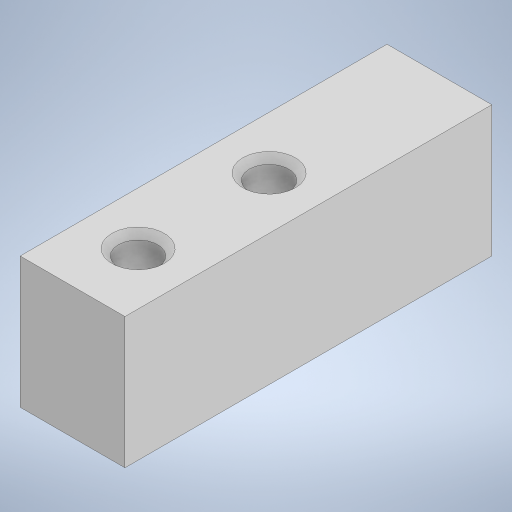
# Autodesk Inventor part: Ограничитель
Saved by Autodesk Inventor 2023 (Build 270158000, 158)
## iProperties
Created: 2022-05-17
Part Number: Ограничитель
Material: Типовые
Document SubType Name: Modeling
Designer: avkap
Density: 1 g/cm^3
Appearance: По умолчанию
Author: avkap
Autodesk Inventor part; units mm, degrees
ref_plane "YZ Plane" through (0, 0, 0) normal (1, 0, 0) x (0, 1, 0)
ref_plane "XZ Plane" through (0, 0, 0) normal (0, 1, 0) x (-1, 0, 0)
ref_plane "XY Plane" through (0, 0, 0) normal (0, 0, 1) x (1, 0, 0)
sketch "Эскиз1" plane through (0, 0, 0) normal (0, 1, 0) x (-1, 0, 0)
  line L0 (0, 0) -> (-8, 0)
  line L1 (-8, 0) -> (-8, -28)
  line L2 (-8, -28) -> (0, -28)
  line L3 (0, -28) -> (0, 0)
  line L4 (-4, 0) -> (-4, -10)
  line L5 (-4, -10) -> (-4, -20)
  line L6 (-4, -20) -> (-4, -15)
  line L7 (-4, 0) -> (-4, -5)
  circle A0 centre (-4, -5) radius 1.5
  circle A1 centre (-4, -15) radius 1.5
  dimension "d0" = 8
  dimension "d1" = 28
  dimension "d2" = 10
  dimension "d3" = 10
  dimension "d4" = 3
  constraints: 16 end point, 3 midpoint, 2 centre point, 2 coincident, 2 parallel, 1 horizontal, 1 perpendicular, 1 point on line, 1 vertical
  measures "d0" distance of L2.end L1.end
  measures "d1" distance of L1.end L0.end
  measures "d2" distance of L4.start L4.end
  measures "d3" distance of L4.end L5.end
  measures "d4" diameter of A0
extrude "Выдавливание1" add sketch "Эскиз1" along normal blind 10
chamfer "Фаска1" distance 0.5 angle 45 4 edges at (5.5, 10, -5) (5.5, 10, -15) (5.5, 0, -15) (5.5, 0, -5)
